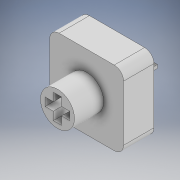
# Autodesk Inventor part: IPC TILS 1 key
Saved by Autodesk Inventor 2022 (Build 260153000, 153)
## iProperties
Created: 2021-12-31
Part Number: IPC TILS 1 key
Material: Generic
Document SubType Name: Modeling
Designer: solor
Density: 1 g/cm^3
Appearance: Default
Author: solor
Autodesk Inventor part; units mm, degrees
ref_plane "YZ Plane" through (0, 0, 0) normal (1, 0, 0) x (0, 1, 0)
ref_plane "XZ Plane" through (0, 0, 0) normal (0, 1, 0) x (-1, 0, 0)
sketch "Sketch1" plane through (0, 0, 0) normal (0, 0, 1) x (1, 0, 0)
  line L0 (14.6962, 12.74) -> (14.6962, 0) construction
  line L1 (10.61, 12.2) -> (1.53, 12.2)
  arc A0 (1.53, 12.2) -> (0, 10.67) centre (1.53, 10.67) ccw
  line L2 (0, 10.67) -> (0, 1.53)
  arc A1 (0, 1.53) -> (1.53, 0) centre (1.53, 1.53) ccw
  line L3 (1.53, 0) -> (10.61, 0)
  arc A2 (10.61, 0) -> (12.14, 1.53) centre (10.61, 1.53) ccw
  arc A3 (12.14, 10.67) -> (10.61, 12.2) centre (10.61, 10.67) ccw
  line L4 (12.14, 10.67) -> (12.14, 1.53)
  point P0 (0, 0)
  point P1 (0, 0)
  dimension "d10" = 12.74
  constraints: 10 end point, 8 point on circle, 4 centre point, 2 vertical, 1 point on line
  measures "d10" distance of L0.start L0.end
ref_plane "Work Plane1" through (0, 0, 5) normal (0, 0, 1) x (1, 0, 0)
sketch "Sketch2" plane through (0, 0, 5) normal (0, 0, 1) x (1, 0, 0)
  line L0 (10.88, 12.74) -> (1.8, 12.74) projected
  line L1 (10.88, 12.74) -> (1.8, 12.74) projected
  arc A0 (1.8, 12.74) -> (0, 10.94) centre (1.8, 10.94) ccw projected
  line L2 (0, 10.94) -> (0, 1.8) projected
  arc A1 (0, 1.8) -> (1.8, 0) centre (1.8, 1.8) ccw projected
  line L3 (1.8, 0) -> (10.88, 0) projected
  arc A2 (10.88, 0) -> (12.68, 1.8) centre (10.88, 1.8) ccw projected
  line L4 (12.68, 1.8) -> (12.68, 10.94) projected
  arc A3 (12.68, 10.94) -> (10.88, 12.74) centre (10.88, 10.94) ccw projected
  circle A4 centre (6.34, 6.37) radius 2.8
  line L5 (5.665, 8.395) -> (7.015, 8.395)
  line L6 (7.015, 4.345) -> (5.665, 4.345)
  line L7 (5.665, 4.345) -> (7.015, 8.395) construction
  line L8 (5.665, 8.395) -> (7.015, 4.345) construction
  line L9 (8.365, 5.695) -> (8.365, 7.045)
  line L10 (4.315, 7.045) -> (4.315, 5.695)
  line L11 (4.315, 5.695) -> (8.365, 7.045) construction
  line L12 (8.365, 5.695) -> (4.315, 7.045) construction
  line L13 (4.315, 5.695) -> (5.665, 5.695)
  line L14 (7.015, 5.695) -> (8.365, 5.695)
  line L15 (5.665, 4.345) -> (5.665, 5.695)
  line L16 (5.665, 7.045) -> (5.665, 8.395)
  line L17 (8.365, 7.045) -> (7.015, 7.045)
  line L18 (5.665, 7.045) -> (4.315, 7.045)
  line L19 (7.015, 8.395) -> (7.015, 7.045)
  line L20 (7.015, 5.695) -> (7.015, 4.345)
  point P0 (0, 0)
  dimension "d3" = 5.6
  dimension "d4" = 4.05
  dimension "d5" = 1.35
  dimension "d6" = 4.05
  dimension "d7" = 1.35
  constraints: 32 end point, 10 parallel, 8 perpendicular, 4 midpoint, 2 vertical, 1 centre point
  measures "d3" diameter of A4
  measures "d4" distance of L6.end L5.start
  measures "d5" distance of L5.start L5.end
  measures "d6" distance of L10.end L9.start
  measures "d7" distance of L9.end L9.start
extrude "Extrusion3" add sketch "Sketch1" along normal blind 5
sketch "Sketch3" plane through (0, 0, 5) normal (0, 0, 1) x (1, 0, 0)
  line L0 (10.61, 12.47) -> (1.53, 12.47)
  line L1 (10.61, 12.47) -> (1.53, 12.47)
  arc A0 (1.53, 12.47) -> (-0.27, 10.67) centre (1.53, 10.67) ccw
  line L2 (-0.27, 10.67) -> (-0.27, 1.53)
  arc A1 (-0.27, 1.53) -> (1.53, -0.27) centre (1.53, 1.53) ccw
  line L3 (1.53, -0.27) -> (10.61, -0.27)
  arc A2 (10.61, -0.27) -> (12.41, 1.53) centre (10.61, 1.53) ccw
  line L4 (12.41, 1.53) -> (12.41, 10.67)
  arc A3 (12.41, 10.67) -> (10.61, 12.47) centre (10.61, 10.67) ccw
  circle A4 centre (6.07, 6.1) radius 2.8
  line L5 (5.395, 8.125) -> (6.745, 8.125)
  line L6 (6.745, 4.075) -> (5.395, 4.075)
  line L7 (5.395, 4.075) -> (6.745, 8.125) construction
  line L8 (5.395, 8.125) -> (6.745, 4.075) construction
  line L9 (8.095, 5.425) -> (8.095, 6.775)
  line L10 (4.045, 6.775) -> (4.045, 5.425)
  line L11 (4.045, 5.425) -> (8.095, 6.775) construction
  line L12 (8.095, 5.425) -> (4.045, 6.775) construction
  line L13 (4.045, 5.425) -> (5.395, 5.425)
  line L14 (6.745, 5.425) -> (8.095, 5.425)
  line L15 (5.395, 4.075) -> (5.395, 5.425)
  line L16 (5.395, 6.775) -> (5.395, 8.125)
  line L17 (8.095, 6.775) -> (6.745, 6.775)
  line L18 (5.395, 6.775) -> (4.045, 6.775)
  line L19 (6.745, 8.125) -> (6.745, 6.775)
  line L20 (6.745, 5.425) -> (6.745, 4.075)
  line L21 (10.61, 12.2) -> (1.53, 12.2) projected
  line L22 (0, 10.67) -> (0, 1.53) projected
  point P0 (0, 0)
  point P1 (-0.27, -0.27)
  point P2 (6.07, 12.2)
  point P3 (0, 6.1)
  point P4 (6.07, 6.1)
  dimension "d14" = 5.6
  dimension "d15" = 4.05
  dimension "d16" = 1.35
  dimension "d17" = 4.05
  dimension "d18" = 1.35
  constraints: 42 end point, 10 parallel, 8 perpendicular, 8 point on circle, 6 midpoint, 5 centre point, 2 vertical
  measures "d14" diameter of A4
  measures "d15" distance of L6.end L5.start
  measures "d16" distance of L5.start L5.end
  measures "d17" distance of L10.end L9.start
  measures "d18" distance of L9.end L9.start
extrude "Extrusion4" add sketch "Sketch3" along normal blind 4.8 contours A4
sketch "Sketch4" plane through (0, 0, 0) normal (0, 0, -1) x (-1, 0, 0)
  line L0 (-1.53, 0) -> (-10.61, 0) projected
  line L1 (-7.4059, 5.3236) -> (-4.7341, 5.3236) construction
  line L2 (-4.7341, 5.3236) -> (-4.7341, 2.2661) construction
  line L3 (-4.7341, 2.2661) -> (-7.4059, 2.2661) construction
  line L4 (-7.4059, 2.2661) -> (-7.4059, 5.3236) construction
  line L5 (-11.8005, 9.9984) -> (-0.3395, 9.9984) construction
  line L6 (-0.3395, 9.9984) -> (-0.3395, 6.8396) construction
  line L7 (-0.3395, 6.8396) -> (-11.8005, 6.8396) construction
  line L8 (-11.8005, 6.8396) -> (-11.8005, 9.9984) construction
  line L9 (-10.8983, 6.894) -> (-10.8983, 9.3632)
  line L10 (-10.8983, 9.3632) -> (-11.8005, 9.3632)
  line L11 (-11.8005, 9.3632) -> (-11.8005, 9.944)
  line L12 (-11.8005, 9.944) -> (-9.23, 9.944)
  line L13 (-9.23, 9.944) -> (-9.23, 9.3632)
  line L14 (-9.23, 9.3632) -> (-10.1321, 9.3632)
  line L15 (-10.1321, 9.3632) -> (-10.1321, 6.894)
  line L16 (-10.1321, 6.894) -> (-10.8983, 6.894)
  line L17 (-7.6506, 7.9568) -> (-9.0075, 7.9568)
  line L18 (-9.0075, 7.9568) -> (-9.0075, 8.5253)
  line L19 (-9.0075, 8.5253) -> (-7.6506, 8.5253)
  line L20 (-7.6506, 8.5253) -> (-7.6506, 7.9568)
  line L21 (-5.5893, 6.894) -> (-7.2304, 6.894)
  line L22 (-7.2304, 6.894) -> (-7.2304, 7.4254)
  line L23 (-7.2304, 7.4254) -> (-6.793, 7.4254)
  line L24 (-6.793, 7.4254) -> (-6.793, 9.4126)
  line L25 (-6.793, 9.4126) -> (-7.2304, 9.4126)
  line L26 (-7.2304, 9.4126) -> (-7.2304, 9.944)
  line L27 (-7.2304, 9.944) -> (-5.5893, 9.944)
  line L28 (-5.5893, 9.944) -> (-5.5893, 9.4126)
  line L29 (-5.5893, 9.4126) -> (-6.0267, 9.4126)
  line L30 (-6.0267, 9.4126) -> (-6.0267, 7.4254)
  line L31 (-6.0267, 7.4254) -> (-5.5893, 7.4254)
  line L32 (-5.5893, 7.4254) -> (-5.5893, 6.894)
  line L33 (-3.046, 6.894) -> (-5.0801, 6.894)
  line L34 (-5.0801, 6.894) -> (-5.0801, 9.944)
  line L35 (-5.0801, 9.944) -> (-4.3139, 9.944)
  line L36 (-4.3139, 9.944) -> (-4.3139, 7.4748)
  line L37 (-4.3139, 7.4748) -> (-3.046, 7.4748)
  line L38 (-3.046, 7.4748) -> (-3.046, 6.894)
  spline S0 degree 2 poles (-1.7385, 6.8396) (-2.0894, 6.8396) (-2.6184, 6.9756) (-2.8457, 7.0744) knots 0 0 0 1 2 2 2
  line L39 (-2.8457, 7.0744) -> (-2.8457, 7.8011)
  line L40 (-2.8457, 7.8011) -> (-2.7765, 7.8011)
  spline S1 degree 2 poles (-2.7765, 7.8011) (-2.5467, 7.6058) (-1.9955, 7.3957) (-1.736, 7.3957) knots 0 0 0 1 2 2 2
  spline S2 degree 2 poles (-1.736, 7.3957) (-1.6692, 7.3957) (-1.4542, 7.4254) (-1.39, 7.4551) knots 0 0 0 1 2 2 2
  spline S3 degree 2 poles (-1.39, 7.4551) (-1.3109, 7.4897) (-1.1996, 7.6157) (-1.1996, 7.717) knots 0 0 0 1 2 2 2
  spline S4 degree 2 poles (-1.1996, 7.717) (-1.1996, 7.8332) (-1.3801, 7.9766) (-1.5037, 8.0087) knots 0 0 0 1 2 2 2
  spline S5 degree 2 poles (-1.5037, 8.0087) (-1.6594, 8.0507) (-2.0128, 8.1224) (-2.1685, 8.1768) knots 0 0 0 1 2 2 2
  spline S6 degree 2 poles (-2.1685, 8.1768) (-2.522, 8.3004) (-2.8284, 8.723) (-2.8284, 9.0394) knots 0 0 0 1 2 2 2
  spline S7 degree 2 poles (-2.8284, 9.0394) (-2.8284, 9.467) (-2.1043, 9.9984) (-1.5605, 9.9984) knots 0 0 0 1 2 2 2
  spline S8 degree 2 poles (-1.5605, 9.9984) (-1.2886, 9.9984) (-0.7498, 9.8871) (-0.5372, 9.7932) knots 0 0 0 1 2 2 2
  line L41 (-0.5372, 9.7932) -> (-0.5372, 9.0962)
  line L42 (-0.5372, 9.0962) -> (-0.604, 9.0962)
  spline S9 degree 2 poles (-0.604, 9.0962) (-0.7745, 9.242) (-1.2639, 9.4422) (-1.521, 9.4422) knots 0 0 0 1 2 2 2
  spline S10 degree 2 poles (-1.521, 9.4422) (-1.6223, 9.4422) (-1.7805, 9.4126) (-1.8695, 9.373) knots 0 0 0 1 2 2 2
  spline S11 degree 2 poles (-1.8695, 9.373) (-1.9411, 9.3409) (-2.0449, 9.2124) (-2.0449, 9.1333) knots 0 0 0 1 2 2 2
  spline S12 degree 2 poles (-2.0449, 9.1333) (-2.0449, 9.0147) (-1.8793, 8.8787) (-1.6421, 8.8243) knots 0 0 0 1 2 2 2
  spline S13 degree 2 poles (-1.6421, 8.8243) (-1.4888, 8.7897) (-1.2046, 8.723) (-1.0415, 8.6662) knots 0 0 0 1 2 2 2
  spline S14 degree 2 poles (-1.0415, 8.6662) (-0.7251, 8.55) (-0.4161, 8.1644) (-0.4161, 7.848) knots 0 0 0 1 2 2 2
  spline S15 degree 2 poles (-0.4161, 7.848) (-0.4161, 7.3933) (-1.1304, 6.8396) (-1.7385, 6.8396) knots 0 0 0 1 2 2 2
  line L43 (-4.9911, 2.2661) -> (-7.0055, 2.2661)
  line L44 (-7.0055, 2.2661) -> (-7.0055, 2.7975)
  line L45 (-7.0055, 2.7975) -> (-6.3629, 2.7975)
  line L46 (-6.3629, 2.7975) -> (-6.3629, 4.4115)
  line L47 (-6.3629, 4.4115) -> (-7.0055, 4.4115)
  line L48 (-7.0055, 4.4115) -> (-7.0055, 4.9083)
  spline S16 degree 2 poles (-7.0055, 4.9083) (-6.8646, 4.9083) (-6.5853, 4.9454) (-6.5013, 4.9849) knots 0 0 0 1 2 2 2
  spline S17 degree 2 poles (-6.5013, 4.9849) (-6.4049, 5.0344) (-6.2962, 5.2) (-6.2863, 5.3236) knots 0 0 0 1 2 2 2
  line L49 (-6.2863, 5.3236) -> (-5.6189, 5.3236)
  line L50 (-5.6189, 5.3236) -> (-5.6189, 2.7975)
  line L51 (-5.6189, 2.7975) -> (-4.9911, 2.7975)
  line L52 (-4.9911, 2.7975) -> (-4.9911, 2.2661)
  point P0 (0, 0)
  point P1 (-6.07, 0)
  point P2 (-6.07, 2.2661)
  point P3 (-6.07, 2.2661)
  point P4 (-6.07, 6.8396)
  point P5 (-6.07, 6.8396)
  constraints: 3 midpoint, 4 other
extrude "Extrusion5" add sketch "Sketch4" along normal blind 0.9
body "Solid2"
